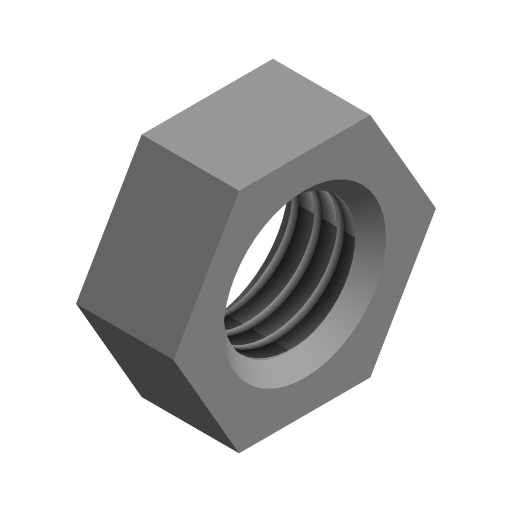
# Autodesk Inventor part: SKNTR4
Saved by Autodesk Inventor 2023.2 (Build 272271000, 271)
## iProperties
Category: PARTsolutions
Company: MISUMI
Part Number: SKNTR4
Material: 일반
Catalog Web Link: www.cadenas.de
Description: LBNR, LBNL, SLBNR, SLBNL, KNTR, KNTL, SKNTR-Nuts
Vendor: MISUMI
Document SubType Name: Modeling
Designer: partserver
Manufacturer: MISUMI
Mass: 0.0855304 g
Surface Area: 1.63532 cm^2
Volume: 0.0855304 cm^3
Density: 1 g/cm^3
Appearance: PSOLRGB-175-175-175
PSOL_IDENT_0: {$CADENAS_DATA\23d-libs\misumi\metric\27_screws_nuts\slbnl.prj},199 {VTYP=3D},{NB=SKNTR4},{LINA=SKNT
PSOL_IDENT_1: R4},{NN=LBNR, LBNL, SLBNR, SLBNL, KNTR, KNTL, SKNTR},{DATE=03.06.2021 03:35:45},{GEOMDATE=05.11.2010
PSOL_IDENT_2: 00:00:00},{VERSION=},{LINEID=30},{WBVAR=TRS,MAT,CS},{WBNUMERIC=}  {NB=SKNTR4},{LINA=SKNTR4},{KT=DUM
PSOL_IDENT_3: MY},{PN=SKNTR4},{TS=KNT},{TRS=R},{MAT=S},{ST=-},{CS=2},{M1=4},{M=4.0},{P=0.70},{B=7.0},{EE=8.1},{T=0
PSOL_IDENT_4: .0},{T1=2.4},{TFX=3.2},{T1FX=2.4},{CALG='1','JIS Class 1','2','JIS Class 3'},{TRSALG= 'R', 'Right-Ha
PSOL_IDENT_5: nd Thread', 'L', 'Left-Hand Thread' },{MATALG= '', 'SWCH Carbon Steel', 'S', '304 Stainless Steel' }
NB: SKNTR4
NN: LBNR, LBNL, SLBNR, SLBNL, KNTR, KNTL, SKNTR
NT: Nuts
NBSYN: $PN.
LINA: SKNTR4
CATALOG: Misumi
PN: SKNTR4
TRS: Right-Hand Thread
MAT: 304 Stainless Steel Equivalent
ST: -
CS: JIS Class 3
M1: 4
P: 0.7
B: 7
EE: 8.1
T: 0
T1: 2.4
SUPPLIER: MISUMI
ARTICLENO: SKNTR4
BOMINFO: SKNTR4
CREATOR: CADENAS GmbH
Title: SKNTR4
Author: Cadenas PARTsolutions
Comments: Nuts
Autodesk Inventor part; units mm, degrees
sketch "Sketch_5" plane through (0, 0, 0) normal (0, 0, 1) x (1, 0, 0)
  line L0 (1.5, 0) -> (-1.5, 0)
  line L1 (-1.5, 0) -> (-1.5, 4.375)
  line L2 (-1.5, 4.375) -> (-1.1031, 5.0625)
  line L3 (-1.1031, 5.0625) -> (1.1031, 5.0625)
  line L4 (1.1031, 5.0625) -> (1.5, 4.375)
  line L5 (1.5, 4.375) -> (1.5, 0)
  line L6 (1.5, 0) -> (-1.5, 0)
  dimension "d8" = 3
  constraints: 14 end point
  measures "d8" distance of L0.start L0.end
revolve "Revolution1" add sketch "Sketch_5" angle 360 about axis through (1.5, 0, 0) along (1, 0, 0)
sketch "Sketch_6" plane through (0, 0, 0) normal (0, 0, 1) x (1, 0, 0)
  line L0 (1.5, 0) -> (-1.5, 0)
  line L1 (-1.5, 0) -> (-1.5, 2.5)
  line L2 (-1.5, 2.5) -> (-1.0262, 2.0262)
  line L3 (-1.0262, 2.0262) -> (1.0263, 2.0262)
  line L4 (1.0263, 2.0262) -> (1.5, 2.5)
  line L5 (1.5, 2.5) -> (1.5, 0)
  line L6 (1.5, 0) -> (-1.5, 0)
  line L7 (0, 2.0262) -> (0, 0)
  line L8 (0, 0) -> (0, 9.277)
  dimension "d10" = 3
  constraints: 18 end point, 2 midpoint, 1 collinear
  measures "d10" distance of L0.start L0.end
revolve "Revolution2" cut sketch "Sketch_6" angle 360 about axis through (1.5, 0, 0) along (1, 0, 0)
thread "Thread1" size "M4x0.7" class "6H" standard "ISO Metric profile" full length
sketch "Sketch_7" plane through (0, 0, 0) normal (1, 0, 0) x (0, 1, 0)
  line L0 (-7, 7) -> (-7, -7)
  line L1 (-7, -7) -> (7, -7)
  line L2 (7, -7) -> (7, 7)
  line L3 (7, 7) -> (-7, 7)
  line L4 (-2.0207, 3.5) -> (-4.0415, 0)
  line L5 (-4.0415, 0) -> (-2.0207, -3.5)
  line L6 (-2.0207, -3.5) -> (2.0207, -3.5)
  line L7 (2.0207, -3.5) -> (4.0415, 0)
  line L8 (4.0415, 0) -> (2.0207, 3.5)
  line L9 (2.0207, 3.5) -> (-2.0207, 3.5)
  constraints: 20 end point
extrude "Extrusion1" cut sketch "Sketch_7" along normal mid plane 3
ref_plane "cp_XY" through (0, 0, 0) normal (1, 0, 0) x (0, 0, -1)
ref_plane "cp_YZ" through (0, 0, 0) normal (0, 0, -1) x (0, 1, 0)
ref_plane "cp_ZX" through (0, 0, 0) normal (0, 1, 0) x (1, 0, 0)
ref_plane "nut_to_screw_XY" through (1.2, 0, 0) normal (1, 0, 0) x (0, 0, -1)
ref_plane "nut_to_screw_YZ" through (1.2, 0, 0) normal (0, 0, -1) x (0, 1, 0)
ref_plane "nut_to_screw_ZX" through (1.2, 0, 0) normal (0, 1, 0) x (1, 0, 0)
body "Solid1"
